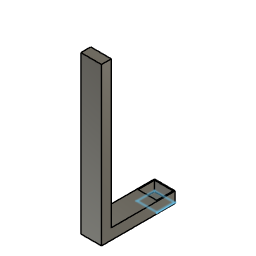
trzymacz v1 (Autodesk Fusion 360 design; units mm, degrees)
Autodesk Fusion 360 part; units mm, degrees
sketch "Szkic1" plane through (0, 0, 0) normal (0, 0, 1) x (1, 0, 0)
  line L0 (-6, -25) -> (-25, -25)
  line L1 (-25, -25) -> (-25, -8.3)
  line L2 (-25, -8.3) -> (-6, -8.3)
  line L3 (-6, -8.3) -> (-6, -25)
  line L4 (-26, -7.3) -> (-5, -7.3)
  line L5 (-5, -7.3) -> (-5, -26)
  line L6 (-5, -26) -> (-26, -26)
  line L7 (-26, -26) -> (-26, -7.3)
  dimension "d1" = 16.7
  dimension "d2" = 19
  dimension "d3" = 1
  dimension "d4" = 1
  dimension "d5" = 1
  dimension "d6" = 1
  constraint horizontal L0
  constraint vertical L1
  constraint horizontal L2
  constraint vertical L3
  constraint horizontal L4
  constraint vertical L5
  constraint horizontal L6
  constraint vertical L7
  measures "d1" distance of L0.end L1.end
  measures "d2" distance of L1.end L2.end
  measures "d3" distance of L1 L7
  measures "d4" distance of L3 L5
  measures "d5" distance of L0 L6
  measures "d6" distance of L2 L4
extrude "Wyciągnięcie proste1" add sketch "Szkic1" along normal blind 10
extrude "Wyciągnięcie proste2" add sketch "Szkic1" against normal blind 1 contours L0 L1 L2 L3 | L4 L5 L6 L7
extrude "Wyciągnięcie proste3" add 1 faces at (-12, -26, 2.6667) along direction (0, -1, 0) blind 46.3
extrude "Wyciągnięcie proste4" add 1 faces at (-12, -72.3, 2.6667) along direction (0, -1, 0) blind 10
sketch "Szkic2" plane through (0, 0, -1) normal (0, 0, -1) x (1, 0, 0)
  line L0 (-26, 82.3) -> (-26, 7.3)
  line L1 (-26, 7.3) -> (-5, 7.3)
  line L2 (-5, 7.3) -> (-5, 82.3)
  line L3 (-5, 82.3) -> (-26, 82.3)
  line L4 (-26, 82.3) -> (-5, 82.3)
  line L5 (-5, 82.3) -> (-5, 72.3)
  line L6 (-5, 72.3) -> (-26, 72.3)
  line L7 (-26, 72.3) -> (-26, 82.3)
  dimension "d15" = 10
  constraint horizontal L4
  constraint vertical L5
  constraint horizontal L6
  constraint vertical L7
  constraint coincident L0.start L3.end
  measures "d15" distance of L0.start L6.end
extrude "Wyciągnięcie proste5" add sketch "Szkic2" against normal blind 160 contours L0 L2 L3 L4 L5 L6 L7
equation "d11 = 65 mm - 18.7 mm"
